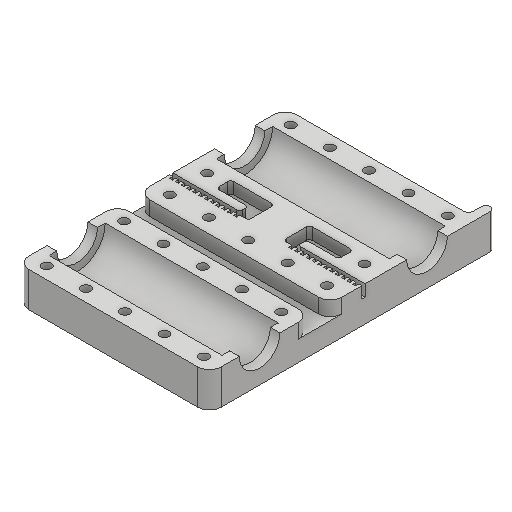
# Autodesk Inventor part: 3DP_ABS_X_Axis_Carriage_Back
Saved by Autodesk Inventor 2026.1 (Build 301233000, 233)
## iProperties
Created: 2016-01-10
Part Number: 3DP_ABS_X_Axis_Carriage_Back
Material: Ogólny
Document SubType Name: Modeling
Designer: Andrzej
Density: 1 g/cm^3
Appearance: Domyślna
Mass: 49.3472 g
Surface Area: 216.395 cm^2
Volume: 49.3472 cm^3
Author: Andrzej
Autodesk Inventor part; units mm, degrees
ref_plane "YZ Plane" through (0, 0, 0) normal (1, 0, 0) x (0, 1, 0)
ref_plane "XZ Plane" through (0, 0, 0) normal (0, 1, 0) x (-1, 0, 0)
ref_plane "XY Plane" through (0, 0, 0) normal (0, 0, 1) x (1, 0, 0)
sketch "Szkic1" plane through (0, 0, 0) normal (0, 0, 1) x (1, 0, 0)
  line L0 (-33, 46) -> (33, 46)
  line L1 (33, 46) -> (33, -46)
  line L2 (33, -46) -> (-33, -46)
  line L3 (-33, -46) -> (-33, 46)
  point P0 (0, 0)
  dimension "d0" = 66
  dimension "d1" = 92
  dimension "d2" = 33
  dimension "d3" = 46
  constraints: 8 end point, 2 parallel, 1 horizontal, 1 perpendicular
  measures "d0" distance of L1.end L2.end
  measures "d1" distance of L0.end L1.end
  measures "d2" distance from line of point (0, 0) L3
  measures "d3" distance from line of L2 point (0, 0)
extrude "Wyciągnięcie proste1" add sketch "Szkic1" along normal blind 12
sketch "Szkic2" plane through (33, -46, 0) normal (1, 0, 0) x (0, 0, -1)
  line L0 (0, 92) -> (0, 0) projected
  line L1 (0, 92) -> (-12, 92) projected
  line L2 (-12, 0) -> (-12, 92) projected
  line L3 (0, 0) -> (-12, 0) projected
  arc A0 (-12, 7.6) -> (-12, 26.9) centre (-12, 17.25) ccw
  arc A1 (-12, 65.1) -> (-12, 84.4) centre (-12, 74.75) ccw
  point P0 (0, 46)
  dimension "d6" = 57.5
  dimension "d7" = 92
  dimension "d8" = 17.25
  dimension "d9" = 12
  dimension "d10" = 19.3
  dimension "d11" = 19.3
  constraints: 4 point on circle, 4 point on line, 2 centre point, 2 coincident
  measures "d6" distance of point (-12, 74.75) point (-12, 17.25)
  measures "d7" distance between parallel lines of L3 L1
  measures "d8" distance from line of L3 point (-12, 17.25)
  measures "d9" distance from line of L0 point (-12, 17.25)
  measures "d10" diameter of A0
  measures "d11" diameter of A1
extrude "Wyciągnięcie proste2" cut sketch "Szkic2" against normal blind 66 contours A1 L2 | L2 A0
sketch "Szkic3" plane through (33, -46, 0) normal (1, 0, 0) x (0, 0, -1)
  arc A0 (-12, 7.6) -> (-12, 26.9) centre (-12, 17.25) ccw projected
  line L0 (-12, 0) -> (-12, 7.6) projected
  line L1 (0, 0) -> (-12, 0) projected
  line L2 (0, 92) -> (0, 0) projected
  line L3 (0, 92) -> (-12, 92) projected
  line L4 (-12, 84.4) -> (-12, 92) projected
  arc A1 (-12, 65.1) -> (-12, 84.4) centre (-12, 74.75) ccw projected
  line L5 (-12, 26.9) -> (-12, 65.1) projected
  line L6 (-12, 7.6) -> (-12, 26.9)
  line L7 (-12, 65.1) -> (-12, 84.4)
  arc A2 (-12, 10.25) -> (-12, 24.25) centre (-12, 17.25) ccw
  arc A3 (-12, 67.75) -> (-12, 81.75) centre (-12, 74.75) ccw
  point P0 (0, 46)
  dimension "d14" = 14
  dimension "d15" = 14
  constraints: 4 end point, 4 point on circle, 4 point on line, 2 centre point, 2 coincident, 1 collinear, 1 vertical
  measures "d14" diameter of A2
  measures "d15" diameter of A3
extrude "Wyciągnięcie proste3" add sketch "Szkic3" against normal blind 3.3 contours L6 A2 A0 | L7 A3 A1
sketch "Szkic4" plane through (-33, -46, 0) normal (-1, 0, 0) x (0, 0, 1)
  arc A0 (12, 26.9) -> (12, 7.6) centre (12, 17.25) ccw projected
  line L0 (12, 65.1) -> (12, 26.9) projected
  arc A1 (12, 84.4) -> (12, 65.1) centre (12, 74.75) ccw projected
  line L1 (12, 92) -> (12, 84.4) projected
  line L2 (0, 92) -> (12, 92) projected
  line L3 (0, 0) -> (0, 92) projected
  line L4 (0, 0) -> (12, 0) projected
  line L5 (12, 7.6) -> (12, 0) projected
  line L6 (12, 24.25) -> (12, 26.9) projected
  arc A2 (12, 26.9) -> (12, 7.6) centre (12, 17.25) ccw projected
  line L7 (12, 7.6) -> (12, 10.25) projected
  arc A3 (12, 24.25) -> (12, 10.25) centre (12, 17.25) ccw projected
  line L8 (12, 81.75) -> (12, 84.4) projected
  arc A4 (12, 84.4) -> (12, 65.1) centre (12, 74.75) ccw projected
  line L9 (12, 65.1) -> (12, 67.75) projected
  arc A5 (12, 81.75) -> (12, 67.75) centre (12, 74.75) ccw projected
  point P0 (0, 46)
extrude "Wyciągnięcie proste4" add sketch "Szkic4" against normal blind 3.3 contours L6 A3 L7 A0 | A1 L8 A5 L9
sketch "Szkic5" plane through (0, 0, 12) normal (0, 0, 1) x (1, 0, 0)
  line L0 (-29.7, -19.1) -> (29.7, -19.1) projected
  line L1 (29.7, -21.75) -> (29.7, -19.1) projected
  line L2 (33, -21.75) -> (29.7, -21.75) projected
  line L3 (33, 21.75) -> (33, -21.75) projected
  line L4 (33, 21.75) -> (29.7, 21.75) projected
  line L5 (29.7, 19.1) -> (29.7, 21.75) projected
  line L6 (29.7, 19.1) -> (-29.7, 19.1) projected
  line L7 (-29.7, 21.75) -> (-29.7, 19.1) projected
  line L8 (-33, 21.75) -> (-29.7, 21.75) projected
  line L9 (-33, 21.75) -> (-33, -21.75) projected
  line L10 (-33, -21.75) -> (-29.7, -21.75) projected
  line L11 (-29.7, -19.1) -> (-29.7, -21.75) projected
  line L12 (33, -11.5) -> (-33, -11.5)
  line L13 (-33, 21.75) -> (-33, -21.75) projected
  line L14 (33, -4.5) -> (-33, -4.5)
  line L15 (-33, -46) -> (33, -46) projected
  line L16 (29.7, -38.4) -> (-29.7, -38.4) projected
  line L17 (33, -11.5) -> (33, -4.5)
  line L18 (-33, -11.5) -> (-33, -4.5)
  point P0 (0, 0)
  dimension "d20" = 7.6
  dimension "d21" = 7
  dimension "d22" = 7.6
  constraints: 8 end point, 4 point on line, 3 perpendicular, 1 collinear
  measures "d20" distance between parallel lines of L12 L0
  measures "d21" distance between parallel lines of L12 L14
  measures "d22" distance between parallel lines of L15 L16
extrude "Wyciągnięcie proste5" cut sketch "Szkic5" against normal blind 5 contours L9 L14 L3 L12
sketch "Szkic6" plane through (0, 0, 12) normal (0, 0, 1) x (1, 0, 0)
  line L0 (33, -35.75) -> (33, -46) projected
  line L1 (33, 21.75) -> (29.7, 21.75) projected
  line L2 (29.7, 19.1) -> (29.7, 21.75) projected
  line L3 (29.7, 19.1) -> (-29.7, 19.1) projected
  line L4 (-29.7, 21.75) -> (-29.7, 19.1) projected
  line L5 (-33, 21.75) -> (-29.7, 21.75) projected
  line L6 (-33, 21.75) -> (-33, -4.5) projected
  line L7 (-33, -4.5) -> (33, -4.5) projected
  line L8 (-33, -46) -> (-33, 46) projected
  line L9 (33, 6.35) -> (32, 6.35)
  line L10 (32, 6.35) -> (32, 5.25)
  line L11 (32, 5.25) -> (31, 5.25)
  line L12 (-33, 6.35) -> (-32, 6.35)
  line L13 (-32, 6.35) -> (-32, 5.25)
  line L14 (-32, 5.25) -> (-31, 5.25)
  line L15 (-31, 5.25) -> (-31, 6.35)
  line L16 (33, 7.45) -> (11, 7.45)
  line L17 (-11, 7.45) -> (-33, 7.45)
  line L18 (6, 7.35) -> (6, 14.35)
  line L19 (7, 15.35) -> (20, 15.35)
  line L20 (21, 14.35) -> (21, 11.35)
  line L21 (20, 10.35) -> (11, 10.35)
  line L22 (10, 9.35) -> (10, 8.45)
  line L23 (-6, 7.35) -> (-6, 14.35)
  line L24 (-7, 15.35) -> (-20, 15.35)
  line L25 (-21, 14.35) -> (-21, 11.35)
  line L26 (-20, 10.35) -> (-11, 10.35)
  line L27 (-10, 9.35) -> (-10, 8.45)
  line L28 (31, 5.25) -> (31, 6.35)
  line L29 (29, 5.25) -> (29, 6.35)
  line L30 (30, 6.35) -> (30, 5.25)
  line L31 (27, 5.25) -> (27, 6.35)
  line L32 (28, 6.35) -> (28, 5.25)
  line L33 (25, 5.25) -> (25, 6.35)
  line L34 (26, 6.35) -> (26, 5.25)
  line L35 (23, 5.25) -> (23, 6.35)
  line L36 (24, 6.35) -> (24, 5.25)
  line L37 (21, 5.25) -> (21, 6.35)
  line L38 (22, 6.35) -> (22, 5.25)
  line L39 (19, 5.25) -> (19, 6.35)
  line L40 (20, 6.35) -> (20, 5.25)
  line L41 (17, 5.25) -> (17, 6.35)
  line L42 (18, 6.35) -> (18, 5.25)
  line L43 (15, 5.25) -> (15, 6.35)
  line L44 (16, 6.35) -> (16, 5.25)
  line L45 (13, 5.25) -> (13, 6.35)
  line L46 (14, 6.35) -> (14, 5.25)
  line L47 (11, 5.25) -> (11, 6.35)
  line L48 (12, 6.35) -> (12, 5.25)
  line L49 (9, 5.25) -> (9, 6.35)
  line L50 (10, 6.35) -> (10, 5.25)
  line L51 (31, 6.35) -> (30, 6.35)
  line L52 (10, 6.35) -> (11, 6.35)
  line L53 (12, 6.35) -> (13, 6.35)
  line L54 (14, 6.35) -> (15, 6.35)
  line L55 (16, 6.35) -> (17, 6.35)
  line L56 (18, 6.35) -> (19, 6.35)
  line L57 (20, 6.35) -> (21, 6.35)
  line L58 (22, 6.35) -> (23, 6.35)
  line L59 (24, 6.35) -> (25, 6.35)
  line L60 (26, 6.35) -> (27, 6.35)
  line L61 (28, 6.35) -> (29, 6.35)
  line L62 (33, 7.45) -> (33, 6.35)
  line L63 (-33, 7.45) -> (-33, 6.35)
  line L64 (9, 6.35) -> (7, 6.35)
  line L65 (-29, 5.25) -> (-29, 6.35)
  line L66 (-30, 6.35) -> (-30, 5.25)
  line L67 (-27, 5.25) -> (-27, 6.35)
  line L68 (-28, 6.35) -> (-28, 5.25)
  line L69 (-25, 5.25) -> (-25, 6.35)
  line L70 (-26, 6.35) -> (-26, 5.25)
  line L71 (-23, 5.25) -> (-23, 6.35)
  line L72 (-24, 6.35) -> (-24, 5.25)
  line L73 (-21, 5.25) -> (-21, 6.35)
  line L74 (-22, 6.35) -> (-22, 5.25)
  line L75 (-19, 5.25) -> (-19, 6.35)
  line L76 (-20, 6.35) -> (-20, 5.25)
  line L77 (-17, 5.25) -> (-17, 6.35)
  line L78 (-18, 6.35) -> (-18, 5.25)
  line L79 (-15, 5.25) -> (-15, 6.35)
  line L80 (-16, 6.35) -> (-16, 5.25)
  line L81 (-13, 5.25) -> (-13, 6.35)
  line L82 (-14, 6.35) -> (-14, 5.25)
  line L83 (-11, 5.25) -> (-11, 6.35)
  line L84 (-12, 6.35) -> (-12, 5.25)
  line L85 (-9, 5.25) -> (-9, 6.35)
  line L86 (-10, 6.35) -> (-10, 5.25)
  line L87 (-31, 6.35) -> (-30, 6.35)
  line L88 (-29, 6.35) -> (-28, 6.35)
  line L89 (-27, 6.35) -> (-26, 6.35)
  line L90 (-25, 6.35) -> (-24, 6.35)
  line L91 (-23, 6.35) -> (-22, 6.35)
  line L92 (-21, 6.35) -> (-20, 6.35)
  line L93 (-19, 6.35) -> (-18, 6.35)
  line L94 (-17, 6.35) -> (-16, 6.35)
  line L95 (-15, 6.35) -> (-14, 6.35)
  line L96 (-13, 6.35) -> (-12, 6.35)
  line L97 (-11, 6.35) -> (-10, 6.35)
  line L98 (-9, 6.35) -> (-7, 6.35)
  arc A0 (-11, 7.45) -> (-10, 8.45) centre (-11, 8.45) ccw
  arc A1 (-7, 6.35) -> (-6, 7.35) centre (-7, 7.35) ccw
  arc A2 (-6, 14.35) -> (-7, 15.35) centre (-7, 14.35) ccw
  arc A3 (-10, 9.35) -> (-11, 10.35) centre (-11, 9.35) ccw
  arc A4 (-20, 15.35) -> (-21, 14.35) centre (-20, 14.35) ccw
  arc A5 (-21, 11.35) -> (-20, 10.35) centre (-20, 11.35) ccw
  arc A6 (6, 7.35) -> (7, 6.35) centre (7, 7.35) ccw
  arc A7 (10, 8.45) -> (11, 7.45) centre (11, 8.45) ccw
  arc A8 (11, 10.35) -> (10, 9.35) centre (11, 9.35) ccw
  arc A9 (7, 15.35) -> (6, 14.35) centre (7, 14.35) ccw
  arc A10 (20, 10.35) -> (21, 11.35) centre (20, 11.35) ccw
  arc A11 (21, 14.35) -> (20, 15.35) centre (20, 14.35) ccw
  line L99 (-30, 5.25) -> (-29, 5.25)
  line L100 (-28, 5.25) -> (-27, 5.25)
  line L101 (-26, 5.25) -> (-25, 5.25)
  line L102 (-24, 5.25) -> (-23, 5.25)
  line L103 (-22, 5.25) -> (-21, 5.25)
  line L104 (-20, 5.25) -> (-19, 5.25)
  line L105 (-18, 5.25) -> (-17, 5.25)
  line L106 (-16, 5.25) -> (-15, 5.25)
  line L107 (-14, 5.25) -> (-13, 5.25)
  line L108 (-12, 5.25) -> (-11, 5.25)
  line L109 (-10, 5.25) -> (-9, 5.25)
  line L110 (30, 5.25) -> (29, 5.25)
  line L111 (28, 5.25) -> (27, 5.25)
  line L112 (26, 5.25) -> (25, 5.25)
  line L113 (24, 5.25) -> (23, 5.25)
  line L114 (22, 5.25) -> (21, 5.25)
  line L115 (20, 5.25) -> (19, 5.25)
  line L116 (18, 5.25) -> (17, 5.25)
  line L117 (16, 5.25) -> (15, 5.25)
  line L118 (14, 5.25) -> (13, 5.25)
  line L119 (12, 5.25) -> (11, 5.25)
  line L120 (10, 5.25) -> (9, 5.25)
  line L121 (33, -11.5) -> (-33, -11.5) projected
  line L122 (-33, -11.5) -> (-33, -21.75) projected
  line L123 (-33, -21.75) -> (-29.7, -21.75) projected
  line L124 (-29.7, -19.1) -> (-29.7, -21.75) projected
  line L125 (-29.7, -19.1) -> (29.7, -19.1) projected
  line L126 (29.7, -21.75) -> (29.7, -19.1) projected
  line L127 (33, -21.75) -> (29.7, -21.75) projected
  line L128 (33, 21.75) -> (33, -4.5) projected
  line L129 (-29.7, 38.4) -> (29.7, 38.4) projected
  line L130 (29.7, 35.75) -> (29.7, 38.4) projected
  line L131 (33, 35.75) -> (29.7, 35.75) projected
  line L132 (33, 35.75) -> (33, 46) projected
  line L133 (33, 46) -> (-33, 46) projected
  line L134 (-33, 46) -> (-33, 35.75) projected
  line L135 (-33, 35.75) -> (-29.7, 35.75) projected
  line L136 (-29.7, 38.4) -> (-29.7, 35.75) projected
  line L137 (29.7, -38.4) -> (-29.7, -38.4) projected
  line L138 (-29.7, -35.75) -> (-29.7, -38.4) projected
  line L139 (-33, -35.75) -> (-29.7, -35.75) projected
  line L140 (-33, -35.75) -> (-33, -46) projected
  line L141 (-33, -46) -> (33, -46) projected
  line L142 (33, -35.75) -> (29.7, -35.75) projected
  line L143 (29.7, -38.4) -> (29.7, -35.75) projected
  line L144 (33, -11.5) -> (33, -21.75) projected
  point P0 (0, 0)
  point P1 (-33, 0.2)
  point P2 (-33, -42)
  point P3 (-33, 42)
  point P4 (10, 7.45)
  point P5 (-10, 7.45)
  point P6 (6, 6.35)
  point P7 (-6, 6.35)
  point P8 (6, 15.35)
  point P9 (21, 15.35)
  point P10 (21, 10.35)
  point P11 (10, 10.35)
  point P12 (-6, 15.35)
  point P13 (-21, 15.35)
  point P14 (-21, 10.35)
  point P15 (-10, 10.35)
  dimension "d27" = 1
  dimension "d29" = 1.1
  dimension "d30" = 1
  dimension "d38" = 1
  dimension "d39" = 1
  dimension "d47" = 4
  dimension "d48" = 4
  dimension "d49" = 9
  dimension "d50" = 15
  dimension "d51" = 5
  dimension "d52" = 9
  dimension "d53" = 15
  dimension "d54" = 5
  dimension "d69" = 1
  dimension "d70" = 1
  dimension "d122" = 1.1
  dimension "d123" = 1.1
  dimension "d124" = 1.1
  constraints: 224 end point, 29 horizontal, 29 point on line, 24 point on circle, 24 tangent, 23 perpendicular, 12 centre point, 10 equal radius, 9 collinear, 6 vertical, 2 parallel
  measures "d27" distance of L9.start L9.end
  measures "d29" distance of L9.end L10.end
  measures "d30" distance of L10.end L11.end
  measures "d38" distance of L12.start L12.end
  measures "d39" distance of L13.end L14.end
  measures "d47" horizontal distance of point (6, 6.35) point (10, 7.45)
  measures "d48" horizontal distance of point (-6, 6.35) point (-10, 7.45)
  measures "d49" distance of point (6, 6.35) point (6, 15.35)
  measures "d50" distance of point (6, 15.35) point (21, 15.35)
  measures "d51" distance of point (21, 15.35) point (21, 10.35)
  measures "d52" distance of point (-6, 6.35) point (-6, 15.35)
  measures "d53" distance of point (-6, 15.35) point (-21, 15.35)
  measures "d54" distance of point (-21, 15.35) point (-21, 10.35)
  measures "d69" radius of A0
  measures "d70" radius of A4
  measures "d122" distance between parallel lines of L87 L17
  measures "d123" distance between parallel lines of L16 L9
  measures "d124" distance of L12.end L13.end
extrude "Wyciągnięcie proste6" cut sketch "Szkic6" against normal blind 4 contours L62 L9 L10 L11 L28 L51 L30 L110 L29 L61 L32 L111 L31 L60 L34 L112 L33 L59 L36 L113 L35 L58 L38 L114 L37 L57 L40 L115 L39 L56 L42 L116 L41 L55 L44 L117 L43 L54 L46 L118 L45 L53 L48 L119 L47 L52 L50 L120 L49 L64 A6 L18 A9 L19 A11 L20 A10 L21 A8 L22 A7 L16 | L6 L17 A0 L27 A3 L26 A5 L25 A4 L24 A2 L23 A1 L98 L85 L109 L86 L97 L83 L108 L84 L96 L81 L107 L82 L95 L79 L106 L80 L94 L77 L105 L78 L93 L75 L104 L76 L92 L73 L103 L74 L91 L71 L102 L72 L90 L69 L101 L70 L89 L67 L100 L68 L88 L65 L99 L66 L87 L15 L14 L13 L12
sketch "Szkic7" plane through (0, 0, 12) normal (0, 0, 1) x (1, 0, 0)
  line L0 (33, -35.75) -> (33, -21.75) projected
  line L1 (-33, -35.75) -> (-33, 7.45) projected
  line L2 (-33, -46) -> (33, -46) projected
  line L3 (29.7, -38.4) -> (-29.7, -38.4) projected
  line L4 (-29.7, -19.1) -> (29.7, -19.1) projected
  line L5 (33, -11.5) -> (-33, -11.5) projected
  line L6 (33, -11.5) -> (33, -21.75) projected
  line L7 (-33, 21.75) -> (-33, -21.75) projected
  line L8 (-33, -4.5) -> (33, -4.5) projected
  line L9 (20, 4.7) -> (19, 4.7) projected
  line L10 (33, 6.35) -> (33, -4.5) projected
  line L11 (-33, 6.35) -> (-33, 7.45) projected
  line L12 (-33, 21.75) -> (-33, 35.75) projected
  line L13 (33, 35.75) -> (33, -21.75) projected
  line L14 (33, 46) -> (-33, 46) projected
  line L15 (-29.7, 38.4) -> (29.7, 38.4) projected
  line L16 (22, 5.25) -> (21, 5.25) projected
  line L17 (33, 21.75) -> (33, 7.45) projected
  line L18 (-33, 21.75) -> (-33, 7.45) projected
  line L19 (-33, 7.45) -> (-11, 7.45) projected
  line L20 (29.7, 19.1) -> (-29.7, 19.1) projected
  line L21 (11, 7.45) -> (33, 7.45) projected
  point P0 (0, 0)
  point P1 (27, -41.9)
  point P2 (13.5, -41.9)
  point P3 (-13.5, -41.9)
  point P4 (-27, -41.9)
  point P5 (33, -42)
  point P6 (-33, -42)
  point P7 (-29, -46)
  point P8 (29, -46)
  point P9 (0, -42)
  point P10 (29, -10.8)
  point P11 (-29, -10.8)
  point P12 (27, -15.3)
  point P13 (13.5, -15.3)
  point P14 (-13.5, -15.3)
  point P15 (-27, -15.3)
  point P16 (0, -15.3)
  point P17 (33, -14.8)
  point P18 (-33, -14.8)
  point P19 (27, 0.375)
  point P20 (13.5, 0.375)
  point P21 (-13.5, 0.375)
  point P22 (-27, 0.375)
  point P23 (-29, -3.8)
  point P24 (29, -3.8)
  point P25 (33, 0.2)
  point P26 (-33, 0.2)
  point P27 (0, 0.375)
  point P28 (27, 41.9)
  point P29 (13.5, 41.9)
  point P30 (0, 41.9)
  point P31 (-13.5, 41.9)
  point P32 (-27, 41.9)
  point P33 (-33, 42)
  point P34 (33, 42)
  point P35 (29, 46)
  point P36 (-29, 46)
  point P37 (27, 13.275)
  point P38 (-27, 13.275)
  point P39 (-33, -11.5)
  dimension "d71" = 13.5
  dimension "d72" = 6
  dimension "d75" = 6
  dimension "d76" = 66
  dimension "d77" = 7.6
  dimension "d78" = 4.1
  dimension "d79" = 4.1
  dimension "d80" = 4.1
  dimension "d81" = 4.1
  dimension "d82" = 13.5
  dimension "d90" = 7.6
  dimension "d91" = 3.8
  dimension "d92" = 3.8
  dimension "d93" = 3.8
  dimension "d94" = 3.8
  dimension "d95" = 3.8
  dimension "d96" = 6
  dimension "d97" = 13.5
  dimension "d98" = 13.5
  dimension "d99" = 6
  dimension "d101" = 4.875
  dimension "d102" = 4.875
  dimension "d104" = 4.875
  dimension "d105" = 4.875
  dimension "d107" = 6
  dimension "d108" = 13.5
  dimension "d109" = 13.5
  dimension "d110" = 6
  dimension "d111" = 4.875
  dimension "d112" = 6
  dimension "d113" = 13.5
  dimension "d114" = 6
  dimension "d115" = 13.5
  dimension "d116" = 7.6
  dimension "d117" = 3.5
  dimension "d118" = 3.5
  dimension "d119" = 3.5
  dimension "d120" = 3.5
  dimension "d121" = 3.5
  dimension "d125" = 9.75
  dimension "d126" = 6
  dimension "d127" = 6
  dimension "d128" = 11.65
  dimension "d129" = 5.825
  dimension "d130" = 5.825
  constraints: 2 other
  measures "d71" distance of point (13.5, -41.9) point (27, -41.9)
  measures "d72" distance from line of point (27, -41.9) L0
  measures "d75" distance from line of L1 point (-27, -41.9)
  measures "d76" distance between parallel lines of L1 L0
  measures "d77" distance between parallel lines of L2 L3
  measures "d78" distance from line of L2 point (27, -41.9)
  measures "d79" distance from line of L2 point (13.5, -41.9)
  measures "d80" distance from line of L2 point (-13.5, -41.9)
  measures "d81" distance from line of L2 point (-27, -41.9)
  measures "d82" distance of point (-27, -41.9) point (-13.5, -41.9)
  measures "d91" distance from line of L4 point (27, -15.3)
  measures "d92" distance from line of L4 point (13.5, -15.3)
  measures "d93" distance from line of L4 point (0, -15.3)
  measures "d94" distance from line of L4 point (-13.5, -15.3)
  measures "d95" distance from line of L4 point (-27, -15.3)
  measures "d96" distance from line of L6 point (27, -15.3)
  measures "d97" distance of point (13.5, -15.3) point (27, -15.3)
  measures "d98" distance of point (-27, -15.3) point (-13.5, -15.3)
  measures "d99" distance from line of L7 point (-27, -15.3)
  measures "d107" distance from line of point (27, 0.375) L10
  measures "d108" distance of point (13.5, 0.375) point (27, 0.375)
  measures "d109" distance of point (-27, 0.375) point (-13.5, 0.375)
  measures "d110" distance from line of L11 point (-27, 0.375)
  measures "d112" distance from line of L12 point (-27, 41.9)
  measures "d113" distance of point (-13.5, 41.9) point (-27, 41.9)
  measures "d114" distance from line of point (27, 41.9) L13
  measures "d115" distance of point (13.5, 41.9) point (27, 41.9)
  measures "d116" distance between parallel lines of L14 L15
  measures "d117" distance from line of L15 point (27, 41.9)
  measures "d118" distance from line of L15 point (13.5, 41.9)
  measures "d119" distance from line of L15 point (0, 41.9)
  measures "d120" distance from line of L15 point (-13.5, 41.9)
  measures "d121" distance from line of L15 point (-27, 41.9)
  measures "d126" distance from line of L17 point (27, 13.275)
  measures "d127" distance from line of L18 point (-27, 13.275)
  measures "d128" distance between parallel lines of L19 L20
  measures "d129" distance from line of L19 point (-27, 13.275)
  measures "d130" distance from line of L21 point (27, 13.275)
hole "Otwór1" at (27, -41.9, 12) at (13.5, -41.9, 12) at (-13.5, -41.9, 12) at (-27, -41.9, 12) at (0, -42, 12) at (27, -15.3, 12) at (13.5, -15.3, 12) at (0, -15.3, 12) at (-13.5, -15.3, 12) at (-27, -15.3, 12) at (27, 0.375, 12) at (13.5, 0.375, 12) at (0, 0.375, 12) at (-13.5, 0.375, 12) at (-27, 0.375, 12) at (13.5, 41.9, 12) at (0, 41.9, 12) at (-13.5, 41.9, 12) at (-27, 41.9, 12) at (27, 41.9, 12) at (-27, 13.275, 12) at (27, 13.275, 12) direction (0, 0, -1) diameter 3.2 end through all
fillet "Zaokrąglenie2" radius 4 6 edges at (-33, -4.5, 9.5) (-33, -11.5, 9.5) (-33, -46, 6) (33, -4.5, 9.5) (33, -11.5, 9.5) (33, -46, 6)
sketch "Szkic8" plane through (0, 0, 0) normal (0, 0, -1) x (-1, 0, 0)
  arc A0 (-33, -42) -> (-29, -46) centre (-29, -42) ccw projected
  line L0 (-29, -46) -> (29, -46) projected
  arc A1 (29, -46) -> (33, -42) centre (29, -42) ccw projected
  line L1 (33, -42) -> (33, 46) projected
  line L2 (33, 46) -> (-33, 46) projected
  line L3 (-33, 46) -> (-33, -42) projected
  circle A2 centre (-27, 13.275) radius 1.6 projected
  circle A3 centre (-27, 41.9) radius 1.6 projected
  circle A4 centre (13.5, 41.9) radius 1.6 projected
  circle A5 centre (-13.5, 41.9) radius 1.6 projected
  circle A6 centre (13.5, 0.375) radius 1.6 projected
  circle A7 centre (-13.5, 0.375) radius 1.6 projected
  circle A8 centre (27, -15.3) radius 1.6 projected
  circle A9 centre (0, -15.3) radius 1.6 projected
  circle A10 centre (-27, -15.3) radius 1.6 projected
  circle A11 centre (27, -41.9) radius 1.6 projected
  circle A12 centre (-13.5, -41.9) radius 1.6 projected
  circle A13 centre (-27, -41.9) radius 1.6 projected
  circle A14 centre (13.5, -41.9) radius 1.6 projected
  circle A15 centre (0, -42) radius 1.6 projected
  circle A16 centre (-13.5, -15.3) radius 1.6 projected
  circle A17 centre (13.5, -15.3) radius 1.6 projected
  circle A18 centre (-27, 0.375) radius 1.6 projected
  circle A19 centre (0, 0.375) radius 1.6 projected
  circle A20 centre (27, 0.375) radius 1.6 projected
  circle A21 centre (0, 41.9) radius 1.6 projected
  circle A22 centre (27, 41.9) radius 1.6 projected
  circle A23 centre (27, 13.275) radius 1.6 projected
  line L4 (-33, 46) -> (-33, 52)
  line L5 (-33, 52) -> (-30, 52)
  line L6 (-30, 52) -> (-30, 46)
  line L7 (-33, 46) -> (33, 46) projected
  line L8 (33, 46) -> (33, 51)
  line L9 (33, 51) -> (23, 51)
  line L10 (23, 51) -> (23, 46)
  line L11 (24.5, 46) -> (24.5, 49.5)
  line L12 (24.5, 49.5) -> (31.5, 49.5)
  line L13 (31.5, 49.5) -> (31.5, 46)
  line L14 (0, 51) -> (-5, 51)
  line L15 (-5, 51) -> (-5, 46)
  line L16 (0, 51) -> (5, 51)
  line L17 (5, 51) -> (5, 46)
  line L18 (3.5, 46) -> (3.5, 49.5)
  line L19 (3.5, 49.5) -> (0, 49.5)
  line L20 (0, 49.5) -> (-3.5, 49.5)
  line L21 (-3.5, 49.5) -> (-3.5, 46)
  line L22 (5, 46) -> (3.5, 46)
  line L23 (33, 46) -> (-33, 46) projected
  line L24 (-3.5, 46) -> (-5, 46)
  line L25 (24.5, 46) -> (23, 46)
  line L26 (33, 46) -> (31.5, 46)
  point P0 (0, 0)
  dimension "d132" = 6
  dimension "d133" = 3
  dimension "d134" = 5
  dimension "d135" = 10
  dimension "d136" = 1.5
  dimension "d137" = 5
  dimension "d138" = 5
  dimension "d139" = 1.5
  constraints: 42 end point, 8 perpendicular, 5 point on line, 4 collinear, 2 vertical, 5 other
  measures "d132" distance of L2.end L4.end
  measures "d133" distance of L4.end L5.end
  measures "d134" distance of L1.end L8.end
  measures "d135" distance of L8.end L9.end
  measures "d136" distance between parallel lines of L9 L12
  measures "d137" distance of L14.start L14.end
  measures "d138" distance of L14.start L16.end
  measures "d139" distance between parallel lines of L16 L19
extrude "Wyciągnięcie proste7" add sketch "Szkic8" against normal blind 12 contours L4 L5 L6 L2
extrude "Wyciągnięcie proste8" add sketch "Szkic8" against normal blind 6 contours L15 L14 L16 L17 L2 L18 L19 L20 L21 | L2 L13 L12 L11 L10 L9 L8
fillet "Zaokrąglenie3" radius 1.5 11 edges at (5, 51, 3) (-5, 51, 3) (-23, 51, 3) (-33, 51, 3) (3.5, 49.5, 3) (-3.5, 49.5, 3) (-24.5, 49.5, 3) (-31.5, 49.5, 3) (30, 52, 6) (33, 52, 6) (30, 46, 6)
chamfer "Faza2" distance 1 angle 45 3 edges at (4.25, 46, 6) (-4.25, 46, 6) (-23.75, 46, 6)
fillet "Zaokrąglenie4" radius 4 1 edges at (-33, 46, 9)
equation "\"d2\" = 0.5 * d0"
equation "\"d3\" = 0.5 * d1"
equation "\"d8\" = -0.5 * d6 + 0.5 * d7"
equation "\"d20\" = d22"
equation "\"d71\" = d82"
equation "\"d72\" = d75"
equation "\"d79\" = d78"
equation "\"d80\" = d79"
equation "\"d81\" = d80"
equation "\"d91\" = 0.5 * d90"
equation "\"d92\" = d91"
equation "\"d93\" = d92"
equation "\"d94\" = d93"
equation "\"d95\" = d94"
equation "\"d102\" = d101"
equation "\"d104\" = d101"
equation "\"d105\" = d101"
equation "\"d111\" = d101"
equation "\"d118\" = d117"
equation "\"d119\" = d117"
equation "\"d120\" = d117"
equation "\"d121\" = d117"
equation "\"d73\" = d71"
